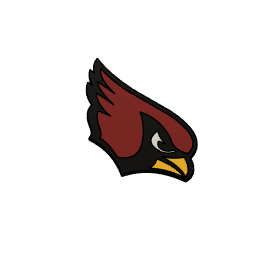
Cardinals (Autodesk Fusion 360 design; units mm, degrees)
Autodesk Fusion 360 part; units mm, degrees
sketch "Sketch1" plane through (0, 0, 0) normal (0, 0, 1) x (1, 0, 0)
  spline S0 degree 2 poles (0, 0) (1.5382, -5.2655) (7.3953, -9.4069) knots 0 0 0 1 1 1
  line L0 (7.3953, -9.4069) -> (3.9639, -9.0223)
  spline S1 degree 2 poles (3.9639, -9.0223) (7.5728, -14.1103) (14.1103, -17.3051) knots 0 0 0 1 1 1
  line L1 (14.1103, -17.3051) -> (10.5605, -16.9797)
  spline S2 degree 2 poles (10.5605, -16.9797) (15.3231, -24.5821) (24.9962, -28.3093) knots 0 0 0 1 1 1
  spline S3 degree 2 poles (24.9962, -28.3093) (25.9724, -34.5214) (34.3439, -40.1123) knots 0 0 0 1 1 1
  spline S4 degree 2 poles (34.3439, -40.1123) (42.3013, -44.6974) (43.2183, -48.8979) knots 0 0 0 1 1 1
  spline S5 degree 2 poles (43.2183, -48.8979) (58.5414, -47.8922) (75.3436, -59.133) knots 0 0 0 1 1 1
  spline S6 degree 2 poles (75.3436, -59.133) (79.3075, -42.9225) (99.8369, -40.9701) knots 0 0 0 1 1 1
  spline S7 degree 2 poles (99.8369, -40.9701) (99.8665, -32.1845) (88.2115, -26.357) knots 0 0 0 1 1 1
  spline S8 degree 2 poles (88.2115, -26.357) (83.4489, -8.1053) (54.5479, -6.1233) knots 0 0 0 1 1 1
  line L2 (54.5479, -6.1233) -> (30.2025, -6.2121)
  spline S9 degree 2 poles (30.2025, -6.2121) (11.6255, -4.9697) (0, 0) knots 0 0 0 1 1 1
  spline S10 degree 2 poles (7.0108, -4.7626) (11.9804, -11.2705) (26.0907, -14.554) knots 0 0 0 1 1 1
  line L3 (26.0907, -14.554) -> (13.3708, -13.4003)
  spline S11 degree 2 poles (13.3708, -13.4003) (18.1333, -17.9559) (32.2141, -21.4169) knots 0 0 0 1 1 1
  line L4 (32.2141, -21.4169) -> (19.4645, -20.2928)
  spline S12 degree 2 poles (19.4645, -20.2928) (26.6232, -27.0965) (37.7162, -28.9601) knots 0 0 0 1 1 1
  line L5 (37.7162, -28.9601) -> (30.9125, -30.025)
  spline S13 degree 2 poles (30.9125, -30.025) (31.5337, -33.4565) (43.2479, -41.0589) knots 0 0 0 1 1 1
  spline S14 degree 2 poles (43.2479, -41.0589) (47.123, -44.3128) (46.3243, -45.1115) knots 0 0 0 1 1 1
  spline S15 degree 2 poles (46.3243, -45.1115) (52.6843, -45.2002) (63.7773, -50.4066) knots 0 0 0 1 1 1
  spline S16 degree 2 poles (63.7773, -50.4066) (74.4266, -44.9636) (59.5768, -29.108) knots 0 0 0 1 1 1
  spline S17 degree 2 poles (59.5768, -29.108) (52.7731, -21.5944) (45.1115, -16.7134) knots 0 0 0 1 1 1
  spline S18 degree 2 poles (45.1115, -16.7134) (56.6778, -13.9624) (71.0839, -22.2156) knots 0 0 0 1 1 1
  spline S19 degree 2 poles (71.0839, -22.2156) (78.4497, -27.7177) (85.1646, -24.9666) knots 0 0 0 1 1 1
  spline S20 degree 2 poles (85.1646, -24.9666) (82.4135, -11.0338) (56.4411, -8.8152) knots 0 0 0 1 1 1
  line L6 (56.4411, -8.8152) -> (28.2206, -8.8152)
  spline S21 degree 2 poles (28.2206, -8.8152) (16.2697, -7.8982) (7.0108, -4.7626) knots 0 0 0 1 1 1
  spline S22 degree 2 poles (7.0108, -4.7626) (11.9804, -11.2705) (26.0907, -14.554) knots 0 0 0 1 1 1
  line L7 (26.0907, -14.554) -> (13.3708, -13.4003)
  spline S23 degree 2 poles (13.3708, -13.4003) (18.1333, -17.9559) (32.2141, -21.4169) knots 0 0 0 1 1 1
  line L8 (32.2141, -21.4169) -> (19.4645, -20.2928)
  spline S24 degree 2 poles (19.4645, -20.2928) (26.6232, -27.0965) (37.7162, -28.9601) knots 0 0 0 1 1 1
  line L9 (37.7162, -28.9601) -> (30.9125, -30.025)
  spline S25 degree 2 poles (30.9125, -30.025) (31.5337, -33.4565) (43.2479, -41.0589) knots 0 0 0 1 1 1
  spline S26 degree 2 poles (43.2479, -41.0589) (47.123, -44.3128) (46.3243, -45.1115) knots 0 0 0 1 1 1
  spline S27 degree 2 poles (46.3243, -45.1115) (52.6843, -45.2002) (63.7773, -50.4066) knots 0 0 0 1 1 1
  spline S28 degree 2 poles (63.7773, -50.4066) (74.4266, -44.9636) (59.5768, -29.108) knots 0 0 0 1 1 1
  spline S29 degree 2 poles (59.5768, -29.108) (52.7731, -21.5944) (45.1115, -16.7134) knots 0 0 0 1 1 1
  spline S30 degree 2 poles (45.1115, -16.7134) (56.6778, -13.9624) (71.0839, -22.2156) knots 0 0 0 1 1 1
  spline S31 degree 2 poles (71.0839, -22.2156) (78.4497, -27.7177) (85.1646, -24.9666) knots 0 0 0 1 1 1
  spline S32 degree 2 poles (85.1646, -24.9666) (82.4135, -11.0338) (56.4411, -8.8152) knots 0 0 0 1 1 1
  line L10 (56.4411, -8.8152) -> (28.2206, -8.8152)
  spline S33 degree 2 poles (28.2206, -8.8152) (16.2697, -7.8982) (7.0108, -4.7626) knots 0 0 0 1 1 1
  spline S34 degree 2 poles (61.8545, -21.4465) (63.3928, -33.4565) (75.1661, -32.8648) knots 0 0 0 1 1 1
  spline S35 degree 2 poles (75.1661, -32.8648) (79.3075, -31.8591) (80.1358, -27.5698) knots 0 0 0 1 1 1
  line L11 (80.1358, -27.5698) -> (78.5384, -27.5698)
  spline S36 degree 2 poles (78.5384, -27.5698) (77.1481, -31.9478) (73.0363, -31.09) knots 0 0 0 1 1 1
  spline S37 degree 2 poles (73.0363, -31.09) (70.5514, -31.0604) (68.1258, -27.4219) knots 0 0 0 1 1 1
  line L12 (68.1258, -27.4219) -> (72.0305, -26.8894)
  spline S38 degree 2 poles (72.0305, -26.8894) (65.1381, -24.73) (61.8545, -21.4465) knots 0 0 0 1 1 1
  spline S39 degree 2 poles (61.8545, -21.4465) (63.3928, -33.4565) (75.1661, -32.8648) knots 0 0 0 1 1 1
  spline S40 degree 2 poles (75.1661, -32.8648) (79.3075, -31.8591) (80.1358, -27.5698) knots 0 0 0 1 1 1
  line L13 (80.1358, -27.5698) -> (78.5384, -27.5698)
  spline S41 degree 2 poles (78.5384, -27.5698) (77.1481, -31.9478) (73.0363, -31.09) knots 0 0 0 1 1 1
  spline S42 degree 2 poles (73.0363, -31.09) (70.5514, -31.0604) (68.1258, -27.4219) knots 0 0 0 1 1 1
  line L14 (68.1258, -27.4219) -> (72.0305, -26.8894)
  spline S43 degree 2 poles (72.0305, -26.8894) (65.1381, -24.73) (61.8545, -21.4465) knots 0 0 0 1 1 1
  spline S44 degree 2 poles (77.651, -38.2782) (89.6314, -36.0892) (97.7071, -40.0531) knots 0 0 0 1 1 1
  spline S45 degree 2 poles (97.7071, -40.0531) (87.4719, -40.4672) (80.6091, -46.2652) knots 0 0 0 1 1 1
  spline S46 degree 3 poles (80.6091, -46.2652) (80.6091, -46.2356) (81.2303, -41.8576) (77.651, -38.2782) knots 0 0 0 0 1 1 1 1
  spline S47 degree 2 poles (77.651, -38.2782) (89.6314, -36.0892) (97.7071, -40.0531) knots 0 0 0 1 1 1
  spline S48 degree 2 poles (97.7071, -40.0531) (87.4719, -40.4672) (80.6091, -46.2652) knots 0 0 0 1 1 1
  spline S49 degree 3 poles (80.6091, -46.2652) (80.6091, -46.2356) (81.2303, -41.8576) (77.651, -38.2782) knots 0 0 0 0 1 1 1 1
  spline S50 degree 2 poles (77.7989, -35.3793) (90.933, -34.8172) (97.7662, -39.1361) knots 0 0 0 1 1 1
  spline S51 degree 3 poles (97.7662, -39.1361) (96.1393, -32.7465) (85.135, -27.7769) (86.0225, -28.2206) knots 0 0 0 0 1 1 1 1
  spline S52 degree 3 poles (86.0225, -28.2206) (86.0225, -28.191) (83.8334, -33.3381) (77.7989, -35.3793) knots 0 0 0 0 1 1 1 1
  spline S53 degree 2 poles (77.7989, -35.3793) (90.933, -34.8172) (97.7662, -39.1361) knots 0 0 0 1 1 1
  spline S54 degree 3 poles (97.7662, -39.1361) (96.1393, -32.7465) (85.135, -27.7769) (86.0225, -28.2206) knots 0 0 0 0 1 1 1 1
  spline S55 degree 3 poles (86.0225, -28.2206) (86.0225, -28.191) (83.8334, -33.3381) (77.7989, -35.3793) knots 0 0 0 0 1 1 1 1
extrude "Extrude1" add sketch "Sketch1" along normal blind 1 contours S44 S45 S46 S47 S48 S49 | S50 S51 S52 S53 S54 S55 makes body 1 at (89.2861, -34.387, 0) makes body 2 at (83.3165, -40.6015, 0)
extrude "Extrude2" add sketch "Sketch1" along normal blind 1 separate body makes body 3
extrude "Extrude3" add sketch "Sketch1" along normal blind 1 separate body contours S34 S35 L11 S36 S37 L12 S38 S39 S40 L13 S41 S42 L14 S43 makes body 4
extrude "Extrude4" add sketch "Sketch1" along normal blind 1 separate body contours S10 L3 S11 L4 S12 L5 S13 S14 S15 S16 S17 S18 S19 S20 L6 S21 S22 L7 S23 L8 S24 L9 S25 S26 S27 S28 S29 S30 S31 S32 L10 S33 makes body 5
named bodies: "yellow1", "yellow2", "black", "white", "red"
